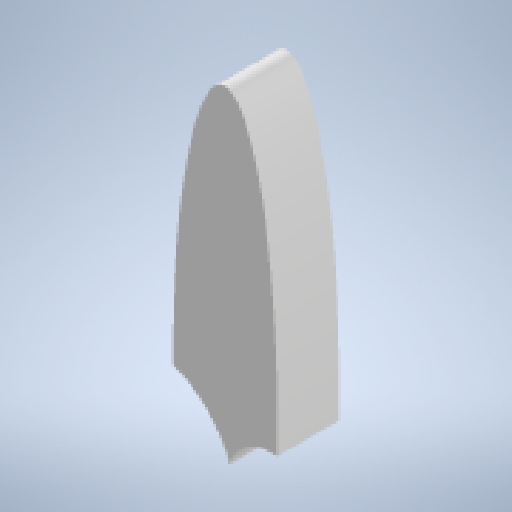
# Autodesk Inventor part: MouthPeach
Saved by Autodesk Inventor 2023 (Build 270158000, 158)
## iProperties
Created: 2022-11-09
Part Number: MouthPeach
Material: Generic
Document SubType Name: Modeling
Designer: reide
Density: 1 g/cm^3
Appearance: Default
Author: reide
Autodesk Inventor part; units mm, degrees
ref_plane "YZ Plane" through (0, 0, 0) normal (1, 0, 0) x (0, 1, 0)
ref_plane "XZ Plane" through (0, 0, 0) normal (0, 1, 0) x (-1, 0, 0)
ref_plane "XY Plane" through (0, 0, 0) normal (0, 0, 1) x (1, 0, 0)
sketch "Sketch1" plane through (0, 0, 0) normal (0, 0, 1) x (1, 0, 0)
  arc A0 (6.4959, 21) -> (2.299, 17.1188) centre (7.4005, 15.8122) ccw projected
  ellipse E0 centre (-2.4643, 17.5498) end of major axis (-7.2277, 17.9807) minor radius 4.1297 (2.1729, 16.4479) -> (2.299, 17.1188) ccw projected
  arc A1 (2.299, 17.1188) -> (2.1729, 16.4479) centre (7.4005, 15.8122) ccw projected
  ellipse E1 centre (-2.4643, 17.5498) end of major axis (2.299, 17.1188) minor radius 4.1297 (2.299, 17.1188) -> (0.0634, 21) ccw projected
  line L0 (6.4959, 21) -> (0.0634, 21) projected
  arc A2 (-52.175, 21) -> (-53.5117, 18.9611) centre (-34.8906, 8.2112) ccw projected
  spline S0 degree 3 poles (-49.4971, 17.2418) (-49.5048, 17.2128) (-49.5128, 17.184) (-49.6432, 16.7374) (-49.8472, 16.3436) (-50.3294, 15.7335) (-50.5829, 15.4969) (-51.1269, 15.1418) (-51.4116, 15.0137) (-51.9673, 14.8843) (-52.2345, 14.868) (-52.6575, 14.9302) (-52.8172, 14.9755) (-52.9676, 15.042) (-53.2518, 15.1676) (-53.5002, 15.3705) (-53.7918, 15.7598) (-53.8781, 15.9145) (-54.1029, 16.4573) (-54.156, 16.8772) (-54.0861, 17.8141) (-53.9112, 18.3281) (-53.5951, 18.8396) (-53.5544, 18.901) (-53.5117, 18.9611) knots -2.04297 -2.04297 -2.04297 -2.04297 -2.033998 -2.033998 -1.903383 -1.903383 -1.8007 -1.8007 -1.70847 -1.70847 -1.629539 -1.629539 -1.580207 -1.580207 -1.580207 -1.486994 -1.486994 -1.434286 -1.434286 -1.31073 -1.31073 -1.152429 -1.152429 -1.130329 -1.130329 -1.130329 -1.130329 projected
  arc A3 (-46.6346, 21) -> (-49.4971, 17.2418) centre (-41.7584, 14.3166) ccw projected
  line L1 (-41.39, 21) -> (-46.6346, 21) projected
  arc A4 (-41.39, 21) -> (-36.9596, 17.2029) centre (-27.9572, 32.1898) ccw projected
  arc A5 (-36.9596, 17.2029) -> (-45.9165, 9.176) centre (-33.54, 4.3762) ccw projected
  arc A6 (-45.9165, 9.176) -> (-47.7565, -7.8721) centre (-18.0941, -2.4502) ccw projected
  arc A7 (-47.7565, -7.8721) -> (-54.7696, -19.1146) centre (-36.7441, -22.5502) ccw projected
  arc A8 (-54.7696, -19.1146) -> (-41.4398, -23.3849) centre (-43.8441, -7.9502) ccw projected
  arc A9 (-41.4398, -23.3849) -> (4.1319, -32.0478) centre (-13.3233, 0.3253) ccw projected
  arc A10 (4.1319, -32.0478) -> (17.2322, -32.7375) centre (11.4815, -17.2068) ccw projected
  arc A11 (17.2322, -32.7375) -> (14.436, -22.6178) centre (2.615, -31.3303) ccw projected
  arc A12 (14.436, -22.6178) -> (17.1111, -9.0721) centre (-4.772, -11.7875) ccw projected
  arc A13 (17.1111, -9.0721) -> (10.587, 12.9757) centre (7.4005, 0.0436) ccw projected
  arc A14 (10.587, 12.9757) -> (8.214, 20) centre (7.4005, 15.8122) ccw projected
  line L2 (8.214, 20) -> (9.5933, 20) projected
  arc A15 (10.5933, 21) -> (9.5933, 20) centre (10.5933, 20) ccw projected
  line L3 (77.7564, 21) -> (10.5933, 21) projected
  line L4 (77.7564, 29.0016) -> (77.7564, 21) projected
  line L5 (-54.0197, 29.0016) -> (77.7564, 29.0016) projected
  arc A16 (-56.0197, 31.0016) -> (-54.0197, 29.0016) centre (-54.0197, 31.0016) ccw projected
  line L6 (-56.0197, 124) -> (-56.0197, 31.0016) projected
  arc A17 (-54.0197, 126) -> (-56.0197, 124) centre (-54.0197, 124) ccw projected
  line L7 (77.7564, 126) -> (-54.0197, 126) projected
  line L8 (77.7564, 134) -> (77.7564, 126) projected
  line L9 (-59.4447, 134) -> (77.7564, 134) projected
  arc A18 (-59.4447, 134) -> (-63.4447, 130) centre (-59.4447, 130) ccw projected
  line L10 (-63.4447, 25) -> (-63.4447, 130) projected
  arc A19 (-63.4447, 25) -> (-59.4447, 21) centre (-59.4447, 25) ccw projected
  line L11 (-52.175, 21) -> (-59.4447, 21) projected
  ellipse E2 centre (-3.2583, 17.5498) end of major axis (-7.6961, 17.5498) minor radius 3.9921 projected
  ellipse E3 centre (-19.8441, -1.5) end of major axis (-22.8441, -1.5) minor radius 2.4928 projected
  arc A20 (-47.0259, -9.6484) -> (-42.4147, -21.5085) centre (93.0716, 37.9945) ccw projected
  arc A21 (-52.5455, -18.26) -> (-42.4147, -21.5085) centre (-41.8746, -2.4026) ccw projected
  arc A22 (-47.0259, -9.6484) -> (-52.5455, -18.26) centre (-34.0085, -24.0666) ccw projected
  arc A23 (1.76, -4.468) -> (0.1559, -5.5) centre (1.5317, -5.8758) ccw projected
  arc A24 (0.1559, -5.5) -> (-1.7702, -3.5257) centre (-2.8441, -6.5) ccw projected
  ellipse E4 centre (0, -3.5) end of major axis (0, 5.5) minor radius 1.7702 (1.76, -4.468) -> (-1.7702, -3.5257) ccw projected
  circle A25 centre (9.1559, -7.9502) radius 2.7388 projected
  circle A26 centre (-12.8441, -6.5) radius 2.8284 projected
  arc A27 (8.3333, -31.4987) -> (14.6255, -25.6953) centre (-5.9975, -9.6484) ccw projected
  arc A28 (15.0836, -31.4172) -> (14.6255, -25.6953) centre (-3.11, -29.9947) ccw projected
  arc A29 (8.3333, -31.4987) -> (15.0836, -31.4172) centre (11.5222, -16.017) ccw projected
  ellipse E5 centre (7.4005, 16.0631) end of major axis (11.4191, 15.7872) minor radius 3.5714 projected
  ellipse E6 centre (15.612, -4.7586) end of major axis (13.0805, -4.7586) minor radius 2.1289 projected
  ellipse E7 centre (0, -3.5) end of major axis (0, 5.05) minor radius 1.6817
  arc A30 (1.672, -4.4196) -> (0.1481, -5.4) centre (1.4551, -5.757) ccw
  arc A31 (0.1481, -5.4) -> (-1.6817, -3.5244) centre (-2.7019, -6.35) ccw
  point P0 (0, 0)
  point P1 (1.672, -4.4196)
  constraints: 4 point on circle, 2 centre point, 1 coincident, 9 other
extrude "Extrusion1" add sketch "Sketch1" along normal blind 2 contours A30 A31 E7
body "Solid1"
